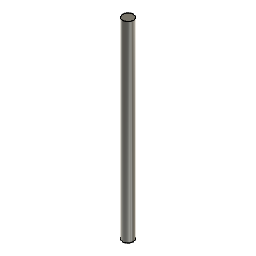
Polín Diámetro 5mm Largo 90mm v1 (Autodesk Fusion 360 design; units mm, degrees)
Autodesk Fusion 360 part; units mm, degrees
cylinder "CilindroPrimitivo1" add diameter 5 height 90 placed x (1, 0, 0) y (0, 1, 0) z (0, 0, 1) at (0, 0, 0)
